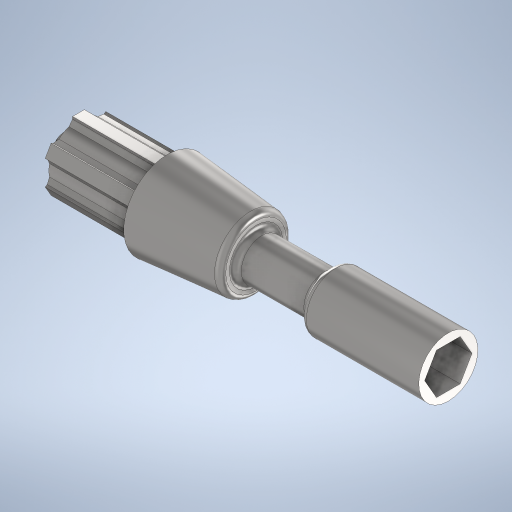
# Autodesk Inventor part: lagnut_screw
Saved by Autodesk Inventor 2023 (Build 270158000, 158)
## iProperties
Created: 2023-11-21
Part Number: lagnut_screw
Material: Steel
Document SubType Name: Modeling
Designer: Beatrice
Density: 7.85 g/cm^3
Appearance: Semi-Polished
Author: Beatrice
Autodesk Inventor part; units mm, degrees
ref_plane "YZ Plane" through (0, 0, 0) normal (1, 0, 0) x (0, 1, 0)
ref_plane "XZ Plane" through (0, 0, 0) normal (0, 1, 0) x (-1, 0, 0)
ref_plane "XY Plane" through (0, 0, 0) normal (0, 0, 1) x (1, 0, 0)
sketch "Sketch1" plane through (0, 0, 0) normal (1, 0, 0) x (0, 1, 0)
  line L0 (1.056781, -0.379193) -> (0.980627, -0.195884)
  line L1 (1.056781, -0.379193) -> (1.12494, -0.418544)
  line L2 (1.12494, -0.418544) -> (0.92494, -0.764955)
  line L3 (0.92494, -0.764955) -> (0.856781, -0.725603)
  line L4 (0.659954, -0.751306) -> (0.856781, -0.725603)
  arc A0 (0.320673, -0.94719) -> (0.659954, -0.751306) centre (0, 0) ccw
  line L5 (0.2, -1.104796) -> (0.320673, -0.94719)
  line L6 (0.2, -1.104796) -> (0.2, -1.183499)
  line L7 (0.2, -1.183499) -> (-0.2, -1.183499)
  line L8 (-0.2, -1.183499) -> (-0.2, -1.104796)
  line L9 (-0.320673, -0.94719) -> (-0.2, -1.104796)
  arc A1 (-0.659954, -0.751306) -> (-0.320673, -0.94719) centre (0, 0) ccw
  line L10 (-0.856781, -0.725603) -> (-0.659954, -0.751306)
  line L11 (-0.856781, -0.725603) -> (-0.92494, -0.764955)
  line L12 (-0.92494, -0.764955) -> (-1.12494, -0.418544)
  line L13 (-1.12494, -0.418544) -> (-1.056781, -0.379193)
  line L14 (-0.980627, -0.195884) -> (-1.056781, -0.379193)
  arc A2 (-0.980627, 0.195884) -> (-0.980627, -0.195884) centre (0, 0) ccw
  line L15 (-1.056781, 0.379193) -> (-0.980627, 0.195884)
  line L16 (-1.056781, 0.379193) -> (-1.12494, 0.418544)
  line L17 (-1.12494, 0.418544) -> (-0.92494, 0.764955)
  line L18 (-0.92494, 0.764955) -> (-0.856781, 0.725603)
  line L19 (-0.659954, 0.751306) -> (-0.856781, 0.725603)
  arc A3 (-0.320673, 0.94719) -> (-0.659954, 0.751306) centre (0, 0) ccw
  line L20 (-0.2, 1.104796) -> (-0.320673, 0.94719)
  line L21 (-0.2, 1.104796) -> (-0.2, 1.183499)
  line L22 (-0.2, 1.183499) -> (0.2, 1.183499)
  line L23 (0.2, 1.183499) -> (0.2, 1.104796)
  line L24 (0.320673, 0.94719) -> (0.2, 1.104796)
  arc A4 (0.659954, 0.751306) -> (0.320673, 0.94719) centre (0, 0) ccw
  line L25 (0.856781, 0.725603) -> (0.659954, 0.751306)
  line L26 (0.856781, 0.725603) -> (0.92494, 0.764955)
  line L27 (0.92494, 0.764955) -> (1.12494, 0.418544)
  line L28 (1.12494, 0.418544) -> (1.056781, 0.379193)
  line L29 (0.980627, 0.195884) -> (1.056781, 0.379193)
  arc A5 (0.980627, -0.195884) -> (0.980627, 0.195884) centre (0, 0) ccw
  circle A6 centre (0, 0) radius 1.469987
  point P0 (0, 0)
  constraints: 60 end point, 12 point on circle, 7 centre point
extrude "Extrusion1" add sketch "Sketch1" against normal blind 3 contours L1 L2 L3 L4 A0 L5 L6 L7 L8 L9 A1 L10 L11 L12 L13 L14 A2 L15 L16 L17 L18 L19 A3 L20 L21 L22 L23 L24 A4 L25 L26 L27 L28 L29 A5 L0
sketch "Sketch1 outline for Extrusion2" plane through (0, 0, 0) normal (1, 0, 0) x (0, 1, 0)
  circle A0 centre (0, 0) radius 1.469987
extrude "Extrusion2" add sketch "Sketch1 outline for Extrusion2" along normal blind 3 draft -5
sketch "Sketch2" plane through (3, 0, 0) normal (1, 0, 0) x (0, 0, -1)
  circle A0 centre (0, 0) radius 0.7
  dimension "d6" = 1.4
  constraints: 1 centre point, 1 coincident
  measures "d6" diameter of A0
extrude "Extrusion3" add sketch "Sketch2" along normal blind 2.5
sketch "Sketch3" plane through (5.5, 0, 0) normal (1, 0, 0) x (0, 0, -1)
  circle A0 centre (0, 0) radius 1
  dimension "d7" = 2
  constraints: 1 centre point, 1 coincident
  measures "d7" diameter of A0
extrude "Extrusion4" add sketch "Sketch3" along normal blind 4
sketch "Sketch4" plane through (9.5, 0, 0) normal (1, 0, 0) x (0, 0, -1)
  circle A0 centre (0, 0) radius 0.8
  line L0 (0, -0.8) -> (-0.69282, -0.4)
  line L1 (-0.69282, -0.4) -> (-0.69282, 0.4)
  line L2 (-0.69282, 0.4) -> (0, 0.8)
  line L3 (0, 0.8) -> (0.69282, 0.4)
  line L4 (0.69282, 0.4) -> (0.69282, -0.4)
  line L5 (0.69282, -0.4) -> (0, -0.8)
  dimension "d10" = 1.6
  constraints: 12 end point, 2 coincident, 1 vertical alignment, 15 other
extrude "Extrusion5" cut sketch "Sketch4" against normal blind 3 contours L4 L5 L0 L1 L2 L3
fillet "Fillet1" radius 0.2 4 edges at (5.5, 0, 1) (3, -1.2075, 0) (3, 0, 0.7) (5.5, 0, 0.7)
sketch "Sketch5" plane through (-3, 0, 0) normal (-1, 0, 0) x (0, 0, 1)
  circle A0 centre (0, 0) radius 0.37
  dimension "d14" = 0.74
  constraints: 1 centre point, 1 coincident
  measures "d14" diameter of A0
extrude "Extrusion6" add sketch "Sketch5" along normal blind 0.5
thread "Thread1" size "M0.8x0.2" class "6g" standard "ANSI Metric M Profile" full length
body "Solid1"
